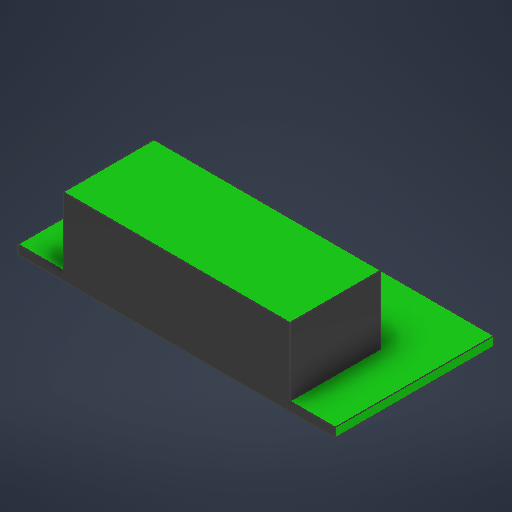
# Autodesk Inventor part: RPpico_dummy
Saved by Autodesk Inventor 2026.1 (Build 301233000, 233)
## iProperties
Created: 2025-12-23
Part Number: RPpico_dummy
Material: Generic
Document SubType Name: Modeling
Designer: emanuel
Density: 1 g/cm^3
Appearance: Default
Author: emanuel
Autodesk Inventor part; units mm, degrees
ref_plane "YZ Plane" through (0, 0, 0) normal (1, 0, 0) x (0, 1, 0)
ref_plane "XZ Plane" through (0, 0, 0) normal (0, 1, 0) x (-1, 0, 0)
ref_plane "XY Plane" through (0, 0, 0) normal (0, 0, 1) x (1, 0, 0)
sketch "Sketch1" plane through (0, 0, 0) normal (0, 1, 0) x (-1, 0, 0)
  line L0 (0, 0) -> (70, 0)
  line L1 (70, 0) -> (70, -50)
  line L2 (70, -50) -> (0, -50)
  line L3 (0, -50) -> (0, 0)
  dimension "d0" = 70
  dimension "d1" = 50
  constraints: 8 end point, 2 parallel, 1 horizontal, 1 perpendicular
  measures "d0" distance of L1.end L2.end
  measures "d1" distance of L0.end L1.end
extrude "Extrusion1" add sketch "Sketch1" along normal blind 2
sketch "Sketch2" plane through (0, 2, 0) normal (0, 1, 0) x (1, 0, 0)
  line L0 (-70, 50) -> (-70, 0) projected
  line L1 (-70, 25) -> (-60, 25)
  line L2 (-60, 25) -> (-60, 15)
  line L3 (-60, 15) -> (-10, 15)
  line L4 (-10, 15) -> (-10, 35)
  line L5 (-10, 35) -> (-60, 35)
  line L6 (-60, 35) -> (-60, 15)
  point P0 (0, 0)
  dimension "d4" = 10
  dimension "d5" = 10
  dimension "d6" = 50
  dimension "d7" = 20
  dimension "d20" = 25
  dimension "d21" = 25
  constraints: 12 end point, 3 midpoint, 2 horizontal, 2 parallel, 2 perpendicular
  measures "d4" distance of L1.start L1.end
  measures "d5" distance of L1.end L2.end
  measures "d6" distance of L5.end L4.end
  measures "d7" distance of L4.end L3.end
  measures "d20" distance of L0.end point (-70, 25)
  measures "d21" distance of L0.start point (-70, 25)
extrude "Extrusion2" add sketch "Sketch2" along normal blind 15
sketch "Sketch3" plane through (0, 2, 0) normal (0, 1, 0) x (1, 0, 0)
  line L0 (0, 50) -> (-70, 50) projected
  line L1 (0, 50) -> (-30, 50)
  line L2 (-30, 50) -> (-30, 45)
  line L3 (-30, 45) -> (0, 45)
  line L4 (0, 45) -> (0, 50)
  line L5 (-70, 50) -> (-70, 0) projected
  line L6 (-70, 0) -> (-40, 0)
  line L7 (-40, 0) -> (-40, 5)
  line L8 (-40, 5) -> (-70, 5)
  line L9 (-70, 5) -> (-70, 0)
  line L10 (-30, 45) -> (-40, 45)
  line L11 (-40, 45) -> (-40, 5)
  line L12 (-40, 5) -> (-30, 5)
  line L13 (-30, 5) -> (-30, 45)
  circle A0 centre (-30, 5) radius 0.5
  circle A1 centre (-40, 5) radius 0.5
  circle A2 centre (-30, 45) radius 0.5
  circle A3 centre (-40, 45) radius 0.5
  point P0 (0, 0)
  dimension "d10" = 30
  dimension "d11" = 5
  dimension "d12" = 30
  dimension "d13" = 5
  dimension "d14" = 1
  dimension "d15" = 1
  dimension "d16" = 1
  dimension "d17" = 1
  constraints: 24 end point, 6 parallel, 4 centre point, 4 coincident, 3 horizontal, 3 perpendicular
  measures "d10" distance of L3.end L2.end
  measures "d11" distance of L2.end L1.end
  measures "d12" distance of L8.end L7.end
  measures "d13" distance of L7.end L6.end
  measures "d14" diameter of A0
  measures "d15" diameter of A1
  measures "d16" diameter of A2
  measures "d17" diameter of A3
extrude "Extrusion3" cut sketch "Sketch3" against normal blind 15 contours A2 L3 L2 | L2 L10 A2 | A2 L13 L3 | L13 A2 L10 | A1 L11 L8 | L8 L7 A1 | A3 L11 L10 | L10 L11 A3 | A0 L12 L13 | L13 L12 A0 | L12 A1 L7 | L11 A1 L12
sketch "Sketch4" plane through (0, 2, 0) normal (0, 1, 0) x (1, 0, 0)
  line L0 (0, 0) -> (0, 50) projected
  line L1 (-70, 50) -> (-70, 0) projected
  line L2 (0, 0) -> (-70, 0)
  line L3 (-70, 0) -> (-70, 15)
  line L4 (-70, 15) -> (0, 15)
  line L5 (0, 15) -> (0, 0)
  dimension "d22" = 15
  constraints: 8 end point, 2 parallel, 1 horizontal, 1 perpendicular, 1 point on line
  measures "d22" distance of L2.end L3.end
extrude "Extrusion4" cut sketch "Sketch4" against normal blind 15
body "Solid1"
